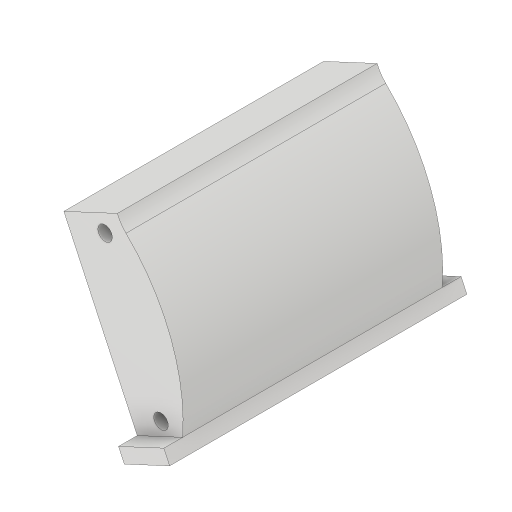
# Autodesk Inventor part: Grip_Side_Down
Saved by Autodesk Inventor 2023.2 (Build 272271000, 271)
## iProperties
Created: 2021-07-28
Part Number: Grip_Side_Down
Material: LCP 플라스틱
Document SubType Name: Modeling
Designer: user
Density: 1.626 g/cm^3
Appearance: 매끄러움 - 흰색
Mass: 7.54033 g
Surface Area: 31.3798 cm^2
Volume: 4.63735 cm^3
Author: user
Autodesk Inventor part; units mm, degrees
ref_plane "YZ Plane" through (0, 0, 0) normal (1, 0, 0) x (0, 1, 0)
ref_plane "XZ Plane" through (0, 0, 0) normal (0, 1, 0) x (-1, 0, 0)
ref_plane "XY Plane" through (0, 0, 0) normal (0, 0, 1) x (1, 0, 0)
sketch "스케치1" plane through (0, 0, 0) normal (0, 0, 1) x (1, 0, 0)
  line L0 (16.9047, -36.2523) -> (26.8143, -31.6314)
  arc A0 (17.3077, -34.3271) -> (17.3407, -34.809) centre (18.2923, -34.5019) ccw
  line L1 (20, -34.809) -> (17.8869, -30.2774)
  line L2 (20, -34.809) -> (25, -34.809) construction
  line L3 (17.8869, -30.2774) -> (26.834, -26.1053)
  arc A1 (26.8143, -31.6314) -> (26.834, -26.1053) centre (-14.2701, -28.7218) ccw
  line L4 (26.834, -26.1053) -> (17.7607, -30.3363)
  arc A2 (16.9047, -36.2523) -> (17.7607, -30.3363) centre (-14.2701, -28.7218) ccw
  line L5 (26.834, -26.1053) -> (16.9047, -36.2523)
  line L6 (17.9253, -30.3598) -> (26.8143, -31.6314)
  circle A3 centre (22.0881, -30.9553) radius 1.6
  point P0 (0, 0)
  point P1 (12.3536, 2.7038)
  point P2 (0.5383, -0.2738)
  dimension "d0" = 5
  dimension "d1" = 115
  dimension "d2" = 90
  dimension "d3" = 3.2
  constraints: 12 end point, 6 point on circle, 5 point on line, 4 centre point, 1 equal length, 1 horizontal, 4 other
  measures "d0" distance of L1.start L1.end
  measures "d1" angle of L2 L1
  measures "d2" angle of L1 L3
  measures "d3" diameter of A3
extrude "돌출1" add sketch "스케치1" along normal blind 56.8
sketch "스케치2" plane through (0, 0, 56.8) normal (0, 0, 1) x (1, 0, 0)
  line L0 (16.9047, -36.2523) -> (26.8143, -31.6314)
  arc A0 (17.3077, -34.3271) -> (18.715, -35.4082) centre (18.2923, -34.5019) ccw
  arc A1 (26.2765, -31.8822) -> (26.8523, -31.032) centre (25.8539, -30.9759) ccw
  line L1 (20, -34.809) -> (17.8869, -30.2774)
  line L2 (20, -34.809) -> (25, -34.809) construction
  line L3 (17.8869, -30.2774) -> (26.834, -26.1053)
  arc A2 (26.8143, -31.6314) -> (12, 3) centre (-14.2701, -28.7218) ccw
  line L4 (26.834, -26.1053) -> (17.7607, -30.3363)
  arc A3 (16.9047, -36.2523) -> (0, 0) centre (-14.2701, -28.7218) ccw
  arc A4 (26.2765, -31.8822) -> (26.8523, -31.032) centre (25.8539, -30.9759) ccw
  circle A5 centre (22.0881, -30.9553) radius 1.6
  line L5 (26.834, -26.1053) -> (22.0881, -30.9553)
  line L6 (19.4569, -33.6442) -> (16.9047, -36.2523)
  line L7 (17.7607, -30.3363) -> (20.5042, -30.7287)
  line L8 (23.6719, -31.1819) -> (26.8143, -31.6314)
  point P0 (12.3536, 2.7038)
  point P1 (0.5383, -0.2738)
  dimension "d6" = 5
  dimension "d7" = 115
  dimension "d8" = 90
  dimension "d9" = 3.2
  constraints: 18 end point, 14 point on circle, 6 centre point, 3 point on line, 1 equal length, 1 horizontal
  measures "d6" distance of L2.start L1.end
  measures "d7" angle of L2 L1
  measures "d8" angle of L1 L3
  measures "d9" diameter of A5
extrude "돌출2" cut sketch "스케치2" against normal up to surface (56.8 mm away) contours A5
sketch "스케치3" plane through (26.8143, -31.6314, 0) normal (0.4226183, -0.9063078, 0) x (0.9063078, 0.4226183, 0)
  line L0 (-10.934, -4.1) -> (0, -4.1)
  line L1 (0, -4.1) -> (0, 60.9)
  line L2 (0, 60.9) -> (-10.934, 60.9)
  line L3 (-10.934, 60.9) -> (-10.934, -4.1)
  line L4 (0, 0) -> (0, 56.8) projected
  line L5 (-10.934, 0) -> (-10.934, 56.8) projected
  dimension "d12" = 65
  dimension "d13" = 4.1
  dimension "d14" = 10.934
  dimension "d15" = 10.934
  dimension "d16" = 10.934
  constraints: 8 end point, 2 parallel, 1 horizontal, 1 perpendicular
  measures "d12" distance between parallel lines of L0 L2
  measures "d13" distance from line of L0 L5.start
  measures "d14" distance between parallel lines of L4 L5
  measures "d15" distance between parallel lines of L1 L3
  measures "d16" distance between parallel lines of L4 L3
extrude "돌출3" add sketch "스케치3" along normal blind 3
sketch "스케치4" plane through (0, 0, 0) normal (0, 0, -1) x (-1, 0, 0)
  circle A0 centre (-6, 44) radius 4.8
  circle A1 centre (-6, 9) radius 4.8
  circle A2 centre (-9.8616, -1.4411) radius 1.6
  circle A3 centre (-22.0881, -30.9553) radius 1.6
  arc A4 (0, 44) -> (-12, 44) centre (-6, 44) ccw
  line L0 (-12, 6.562) -> (-12, 44)
  arc A5 (-14.4262, 0.8233) -> (-12, 6.562) centre (-20, 6.562) ccw
  arc A6 (-14.4262, 0.8233) -> (-26.8143, -31.6314) centre (14.2701, -28.7218) ccw
  line L1 (-16.9047, -36.2523) -> (-26.8143, -31.6314)
  line L2 (-16.9047, -36.2523) -> (0, 0)
  line L3 (0, 44) -> (0, 0)
  line L4 (-16.9047, -36.2523) -> (-26.8143, -31.6314) projected
  line L5 (-26.8143, -31.6314) -> (-28.0821, -34.3503) projected
  line L6 (-18.1726, -38.9712) -> (-28.0821, -34.3503) projected
  line L7 (-16.9047, -36.2523) -> (-18.1726, -38.9712) projected
  circle A7 centre (-22.0881, -30.9553) radius 1.6 projected
  line L8 (-16.9047, -36.2523) -> (-26.8143, -31.6314) projected
  arc A8 (-17.7607, -30.3363) -> (-16.9047, -36.2523) centre (14.2701, -28.7218) ccw projected
  line L9 (-26.834, -26.1053) -> (-17.7607, -30.3363) projected
  arc A9 (-26.834, -26.1053) -> (-26.8143, -31.6314) centre (14.2701, -28.7218) ccw projected
  line L10 (-16.9047, -36.2523) -> (-26.8143, -31.6314) projected
  line L11 (-21.8595, -33.9419) -> (-5.8, 0.4978) construction
  line L12 (-5.8, 0.4978) -> (-0.8452, -1.8126)
  line L13 (-5.8, 0.4978) -> (-12.5505, 3.6456)
  point P0 (0, 0)
  point P1 (0, 0)
  point P2 (-17.7151, -2.7731)
  dimension "d19" = 38
  constraints: 14 end point, 8 point on circle, 7 centre point, 1 collinear, 1 midpoint, 1 parallel, 1 perpendicular, 1 point on line
  measures "d19" distance of L11.start L11.end
extrude "돌출4" add sketch "스케치4" against normal up to surface (56.8 mm away) contours L2 A8 L9 A6 A5 L13 L12
sketch "스케치8" plane through (16.9047, -36.2523, -4.1) normal (-0.9063078, -0.4226183, 0) x (0, 0, 1)
  line L0 (4.1, 38) -> (60.9, 38) projected
  line L1 (4.1, 0) -> (4.1, 38) projected
  line L2 (65, 0) -> (60.9, 0) projected
  line L3 (0, 0) -> (0, -3) projected
  line L4 (65, -3) -> (0, -3) projected
  line L5 (65, 0) -> (65, -3) projected
  line L6 (4.1, 0) -> (0, 0) projected
  line L7 (60.9, 0) -> (60.9, 38) projected
  line L8 (4.1, 0) -> (4.1, 34.6494) projected
  line L9 (61.1, 38) -> (4.1, 38)
  line L10 (4.1, 38) -> (4.1, 0)
  line L11 (4.1, 0) -> (61.1, 0)
  line L12 (61.1, 0) -> (61.1, 38)
  line L13 (4.1, 38) -> (61.1, 38) projected
  line L14 (32.6, 38) -> (32.6, 19)
  line L15 (60.9, 0) -> (60.9, 38) projected
  line L16 (60.9, 19.0005) -> (4.1, 19)
  line L17 (57.6, 34) -> (7.6, 34)
  line L18 (7.6, 34) -> (7.6, 4)
  line L19 (7.6, 4) -> (57.6, 4)
  line L20 (57.6, 4) -> (57.6, 34)
  line L21 (57.6, 34) -> (7.6, 4) construction
  line L22 (7.6, 34) -> (57.6, 4) construction
  point P0 (4.1, 40)
  dimension "d37" = 50
  dimension "d38" = 30
  constraints: 24 end point, 4 midpoint, 4 parallel, 2 horizontal, 2 perpendicular, 1 vertical, 2 other
  measures "d37" distance of L19.end L18.end
  measures "d38" distance of L18.end L17.end
extrude "돌출7" cut sketch "스케치8" against normal blind 3 contours L17 L20 L16 L14 | L14 L16 L18 L17 | L16 L20 L19 L18
equation "\"d15\" = d14"
equation "\"d16\" = d14"
